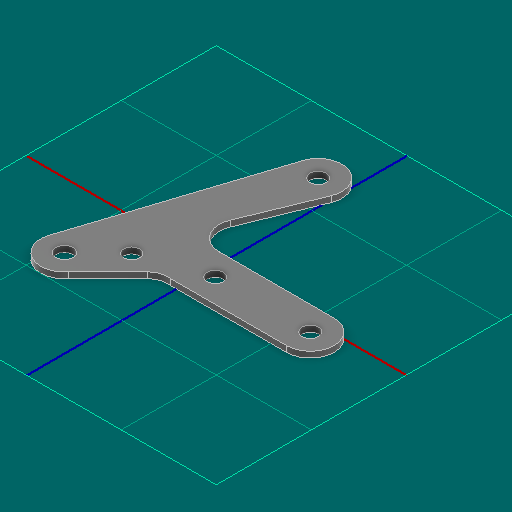
# Autodesk Inventor part: join-gusset_offset
Saved by Autodesk Inventor 2025 (Build 290162000, 162)
## iProperties
Created: 2024-08-11
Part Number: join-gusset_offset
Material: Acetal Resin, Black
Document SubType Name: Sheet Metal
Designer: averey
Density: 1.425 g/cm^3
Sheet Metal Rule: Default
Appearance: Smooth - Black
d0: 0.500 in
Author: averey
Autodesk Inventor part; units mm, degrees
ref_plane "YZ Plane" through (0, 0, 0) normal (1, 0, 0) x (0, 1, 0)
ref_plane "XZ Plane" through (0, 0, 0) normal (0, 1, 0) x (-1, 0, 0)
ref_plane "XY Plane" through (0, 0, 0) normal (0, 0, 1) x (1, 0, 0)
sketch "main" plane through (0, 0, 0) normal (0, 0, 1) x (1, 0, 0)
  circle A0 centre (38.7007, 32.2161) radius 2.3114
  circle A1 centre (29.7205, 23.2358) radius 2.3114
  circle A2 centre (13.1029, 17.5349) radius 2.1844
  circle A3 centre (22.281, -19.1287) radius 2.1844
  circle A4 centre (22.281, -19.1287) radius 6.35
  spline S0 degree 3 poles (34.2106, 36.7062) (34.5464, 37.0421) (35.2145, 37.7033) (36.4253, 38.4715) (37.8969, 38.8878) (39.5045, 38.8877) (40.9769, 38.4718) (42.187, 37.7033) (42.855, 37.0421) (43.1908, 36.7062) knots 0 0 0 0 0.123366 0.246731 0.370097 0.493463 0.616828 0.740194 0.86356 0.86356 0.86356 0.86356
  spline S1 degree 3 poles (43.1908, 36.7062) (43.5267, 36.3703) (44.188, 35.7023) (44.9562, 34.4914) (45.3725, 33.0199) (45.3723, 31.4123) (44.9564, 29.9399) (44.1879, 28.7298) (43.5267, 28.0618) (43.1908, 27.7259) knots 0 0 0 0 0.123366 0.246731 0.370097 0.493463 0.616828 0.740194 0.86356 0.86356 0.86356 0.86356
  line L0 (28.3198, -21.092) -> (45.0845, 30.4731)
  line L1 (16.2421, -17.1653) -> (28.0767, 19.2357)
  line L2 (24.0195, 11.1849) -> (0.4029, 11.1849)
  spline S2 degree 3 poles (28.5097, 13.0448) (28.2578, 12.7929) (27.7518, 12.2921) (26.7458, 11.6097) (25.4482, 11.197) (24.4945, 11.1849) (24.0195, 11.1849) knots 0 0 0 0 0.214286 0.428571 0.714286 1 1 1 1
  point P0 (28.3293, 11.5879)
  dimension "d0" = 12.7
  measures "d0" diameter of A4
sketch "Sketch1" plane through (0, 0, 0) normal (0, 1, 0) x (-1, 0, 0)
  circle A0 centre (21.6209, 18.9442) radius 2.3114
  circle A1 centre (-4.1584, 4.4483) radius 2.1844
  circle A2 centre (5.0197, -32.2153) radius 2.1844
  arc A3 (-0.8574, -29.8106) -> (11.0596, -34.1752) centre (5.0197, -32.2153) ccw
  line L0 (11.0596, -34.1752) -> (27.6609, 16.9843)
  line L1 (-0.8574, -29.8106) -> (6.9797, -10.6563)
  line L2 (1.1026, -1.9017) -> (-29.5584, -1.9017)
  line L3 (6.1274, 12.3495) -> (16.5681, 22.7902)
  spline S0 degree 3 poles (1.4978, 10.7983) (1.9738, 10.7652) (2.9304, 10.7109) (4.2596, 11.0342) (5.3155, 11.648) (5.8574, 12.1146) (6.1274, 12.3495) knots 0 0 0 0 0.285714 0.571429 0.785714 1 1 1 1
  line L4 (-16.8584, 10.7983) -> (1.4978, 10.7983)
  arc A4 (6.9797, -10.6563) -> (1.1026, -1.9017) centre (1.1026, -8.2517) ccw
  line L5 (-16.8584, 10.7983) -> (-29.5584, 10.7983)
  circle A5 centre (-29.5584, 4.4483) radius 2.1844
  arc A6 (27.6609, 16.9843) -> (16.5681, 22.7902) centre (21.6209, 18.9442) ccw
  arc A7 (-29.5584, 10.7983) -> (-29.5584, -1.9017) centre (-29.5584, 4.4483) ccw
  circle A8 centre (12.4592, 10.1492) radius 2.0955
  line L6 (12.3751, 10.0685) -> (21.6209, 18.9442)
  line L7 (15.0275, 12.7176) -> (12.4592, 10.1492)
  dimension "d2" = 12.7
  dimension "d3" = 6.35
  dimension "d10" = 6.35
  dimension "d11" = 3.6322
  dimension "d12" = 12.7
  constraints: 16 end point, 9 centre point, 8 point on circle, 5 tangent, 4 coincident, 2 horizontal, 1 point on line, 6 other
  measures "d2" diameter of A3
  measures "d3" radius of A4
  measures "d10" radius of A6
  measures "d11" distance of L7.start L7.end
  measures "d12" distance of A0.centre A8.centre
extrude "Extrusion1" add sketch "Sketch1" along normal blind 1.5875
equation "\"BendRadius\" = Thickness"
equation "\"BendReliefWidth\" = Thickness"
equation "\"BendReliefDepth\" = 0.5 * Thickness"
equation "\"CornerReliefSize\" = 4 * Thickness"
equation "\"MinimumRemnant\" = 2 * Thickness"
equation "\"TransitionRadius\" = BendRadius"
equation "\"JacobiRadiusSize\" = BendRadius"
equation "\"GapSize\" = Thickness"
equation "\"Thickness\" = 3.048"
body "Solid1"
